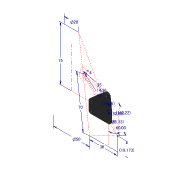
# Autodesk Inventor part: COXA_YAW_SERVO_BASE
Saved by Autodesk Inventor 2019.4 (Build 234330000, 330)
## iProperties
Created: 2019-10-21
Part Number: COXA_YAW_SERVO_BASE
Material: 一般
Document SubType Name: Modeling
Designer: y6tada
Density: 1 g/cm^3
Appearance: Black 80
Author: y6tada
Autodesk Inventor part; units mm, degrees
ref_plane "YZ Plane" through (0, 0, 0) normal (1, 0, 0) x (0, 1, 0)
ref_plane "XZ Plane" through (0, 0, 0) normal (0, 1, 0) x (-1, 0, 0)
ref_plane "XY Plane" through (0, 0, 0) normal (0, 0, 1) x (1, 0, 0)
sketch "スケッチ1" plane through (0, 0, 0) normal (0, 0, 1) x (1, 0, 0)
  line L0 (10, 75) -> (16.2273, 28.555) construction
  line L1 (16.2273, 28.555) -> (51.0067, 0) construction
  line L2 (51.0067, 0) -> (10, 75) construction
  line L3 (51.0067, 0) -> (63, -21.9354) construction
  line L4 (63, -21.9354) -> (25, -36.8749) construction
  line L5 (0, 0) -> (0, 56.2963) construction
  line L6 (0, 0) -> (51.0067, 0) construction
  line L7 (16.2273, 28.555) -> (50.1611, 19.9821) construction
  line L8 (50.1611, 19.9821) -> (51.0067, 0) construction
  arc A0 (21.2901, 31.2723) -> (19.3921, 23.7592) centre (50.1611, 19.9821) ccw construction
  arc A1 (13.8396, 34.1859) -> (11.4517, 24.7339) centre (50.1611, 19.9821) ccw construction
  arc A2 (11.4517, 24.7339) -> (19.3921, 23.7592) centre (15.4219, 24.2465) ccw construction
  arc A3 (21.2901, 31.2723) -> (13.8396, 34.1859) centre (17.5649, 32.7291) ccw construction
  line L9 (15.4219, 24.2465) -> (50.1611, 19.9821) construction
  line L10 (50.1611, 19.9821) -> (17.5649, 32.7291) construction
  arc A4 (17.5649, 32.7291) -> (15.4219, 24.2465) centre (50.1611, 19.9821) ccw construction
  line L11 (16.2273, 28.555) -> (61.5646, -21.7031) construction
  line L12 (61.5646, -21.7031) -> (67.6266, 18.6756) construction
  line L13 (67.6266, 18.6756) -> (51.0067, 0) construction
  arc A5 (48.5023, 0.051) -> (53.4978, 0.2624) centre (50.1611, 19.9821) ccw construction
  line L14 (50.1611, 19.9821) -> (48.5023, 0.051) construction
  line L15 (53.4978, 0.2624) -> (50.1611, 19.9821) construction
  circle A6 centre (51.0067, 0) radius 2.5 construction
  line L16 (51.0067, 0) -> (51.0067, -39.6994) construction
  line L17 (17.5649, 32.7291) -> (25, -36.8749) construction
  dimension "d0" = 20
  dimension "d1" = 50
  dimension "d3" = 25
  dimension "d4" = 38
  dimension "d5" = 75
  dimension "d6" = 45
  dimension "d12" = 4
  dimension "d22" = 20
  dimension "d41" = 35
  dimension "d42" = 60
  dimension "d43" = 92.423
  dimension "d44" = 61.332
  dimension "d47" = 5
  dimension "d48" = 14.361
  dimension "d49" = 14.36
  dimension "d50" = 138.333
  dimension "d51" = 14.9395
  dimension "d52" = 70
  constraints: 36 end point, 15 point on circle, 7 centre point, 4 coincident, 4 tangent, 2 equal length, 2 point on line, 2 symmetric about line, 2 vertical, 1 horizontal
  measures "d0" diameter of L0.start L5
  measures "d1" diameter of L4.end L5
  measures "d3" distance of L1.end L3.end
  measures "d4" horizontal distance of L3.end L4.end
  measures "d5" distance from line of L6 L0.start
  measures "d6" distance of L0.end L1.end
  measures "d12" radius of A3
  measures "d22" distance of L7.end L1.end
  measures "d41" distance of L0.end L7.end
  measures "d42" angle of L4 L12
  measures "d43" angle of L8 L6
  measures "d44" angle of L3 L6
  measures "d47" diameter of A6
  measures "d48" angle of L15 L14
  measures "d49" angle of L9 L10
  measures "d50" angle of L16 L13
  measures "d51" vertical distance of L3.end L4.end
  measures "d52" distance of L10.end L4.end
sketch "スケッチ2" plane through (0, 0, 0) normal (0, 0, 1) x (1, 0, 0)
  arc A0 (54.1384, 20.4075) -> (47.5443, 23.0074) centre (50.1611, 19.9821) ccw
  line L0 (29, 3) -> (53, 3) construction
  line L1 (53, 3) -> (53, -9) construction
  line L2 (53, -9) -> (29, -9) construction
  line L3 (29, -9) -> (29, 3) construction
  line L4 (25, 10.1673) -> (25, -48.9437) construction
  line L5 (56, 3) -> (56, -9)
  line L6 (53, -12) -> (29, -12)
  line L7 (26, -9) -> (26, 3)
  arc A1 (26, -9) -> (29, -12) centre (29, -9) ccw
  arc A2 (27.0374, 5.2689) -> (26, 3) centre (29, 3) ccw
  arc A3 (53, -12) -> (56, -9) centre (53, -9) ccw
  line L8 (0, 0) -> (0, -59.5537) construction
  line L9 (10.6628, -3) -> (66.9205, -3) construction
  line L10 (56, 3) -> (54.1384, 20.4075)
  line L11 (27.0374, 5.2689) -> (47.5443, 23.0074)
  dimension "d16" = 24
  dimension "d17" = 4
  dimension "d18" = 12
  dimension "d19" = 3
  dimension "d20" = 50
  dimension "d21" = 3
  dimension "d23" = 4
  constraints: 24 end point, 8 point on circle, 8 tangent, 4 centre point, 3 coincident, 3 horizontal, 3 parallel, 3 vertical, 2 equal radius, 1 perpendicular, 1 other
  measures "d16" distance of L1.end L2.end
  measures "d17" distance between parallel lines of L3 L4
  measures "d18" distance of L2.end L0.start
  measures "d19" radius of A1
  measures "d20" diameter of L4 L8
  measures "d21" distance from line of L8.start L9
  measures "d23" radius of A0
extrude "押し出し1" add sketch "スケッチ2" along normal blind 2
hole "穴1" at (50.1611, 19.9821, 0) direction (0, 0, 1) diameter 3 end through all
hole "穴2" at (53, 3, 0) at (29, 3, 0) at (29, -9, 0) at (53, -9, 0) direction (0, 0, 1) diameter 2.5 end through all
